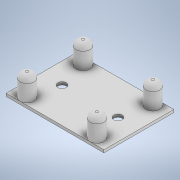
# Autodesk Inventor part: sensor color
Saved by Autodesk Inventor 2021 (Build 250183000, 183)
## iProperties
Created: 2022-05-07
Part Number: sensor color
Material: Genérico
Document SubType Name: Modeling
Designer: uriel
Density: 1 g/cm^3
Appearance: Valor por defecto
Author: uriel
Autodesk Inventor part; units mm, degrees
ref_plane "YZ Plane" through (0, 0, 0) normal (1, 0, 0) x (0, 1, 0)
ref_plane "XZ Plane" through (0, 0, 0) normal (0, 1, 0) x (-1, 0, 0)
ref_plane "XY Plane" through (0, 0, 0) normal (0, 0, 1) x (1, 0, 0)
sketch "Boceto1" plane through (0, 0, 0) normal (0, 1, 0) x (-1, 0, 0)
  line L0 (0, 0) -> (35, 0)
  line L1 (35, 0) -> (35, 25)
  line L2 (35, 25) -> (0, 25)
  line L3 (0, 25) -> (0, 0)
  dimension "d0" = 35
  dimension "d1" = 25
  constraints: 8 end point, 2 parallel, 1 horizontal, 1 perpendicular
  measures "d0" distance of L2.end L1.end
  measures "d1" distance of L0.end L1.end
extrude "Extrusión1" add sketch "Boceto1" along normal blind 1
sketch "Boceto2" plane through (0, 1, 0) normal (0, 1, 0) x (1, 0, 0)
  line L0 (-35, 0) -> (-35, -25) projected
  line L1 (-35, -25) -> (0, -25) projected
  line L2 (0, -25) -> (0, 0) projected
  line L3 (0, 0) -> (-35, 0) projected
  line L4 (-35, -25) -> (0, -25) projected
  line L5 (0, 0) -> (-35, 0) projected
  circle A0 centre (-27.5, -12.5) radius 1.5
  circle A1 centre (-7.5, -12.5) radius 1.5
  line L6 (-35, 0) -> (-35, -25) projected
  line L7 (-35, -25) -> (0, -25) projected
  line L8 (0, -25) -> (0, 0) projected
  line L9 (0, 0) -> (-35, 0) projected
  dimension "d5" = 3
  constraints: 2 centre point
  measures "d5" diameter of A0
extrude "Extrusión2" cut sketch "Boceto2" against normal blind 1 contours A0 | A1
sketch "Boceto3" plane through (0, 1, 0) normal (0, 1, 0) x (1, 0, 0)
  line L0 (-35, -25) -> (0, -25) projected
  line L1 (0, -25) -> (-5, -25)
  line L2 (-5, -25) -> (-5, -22.5)
  circle A0 centre (-5, -22.5) radius 2.5
  line L3 (-35, 0) -> (-35, -25) projected
  line L4 (-17.5, -25) -> (-17.5, 0)
  line L5 (0, 0) -> (-35, 0) projected
  line L6 (-35, 0) -> (-35, -25) projected
  line L7 (-35, -12.5) -> (0, -12.5)
  line L8 (0, -25) -> (0, 0) projected
  circle A1 centre (-30, -22.5) radius 2.5
  line L9 (0, -12.5) -> (-35, -12.5)
  circle A2 centre (-5, -2.5) radius 2.5
  circle A3 centre (-30, -2.5) radius 2.5
  dimension "d8" = 5
  dimension "d9" = 2.5
  dimension "d10" = 5
  constraints: 10 end point, 5 symmetric about line, 4 centre point, 4 midpoint, 1 coincident, 1 perpendicular, 1 point on line, 3 other
  measures "d8" distance of L0.end L1.end
  measures "d9" distance of L1.end L2.end
  measures "d10" diameter of A0
extrude "Extrusión3" add sketch "Boceto3" along normal blind 8 contours A0 | A1 | A3 | A2
fillet "Empalme1" radius 2 4 edges at (-32.5, 9, 22.5) (-32.5, 9, 2.5) (-7.5, 9, 2.5) (-7.5, 9, 22.5)
